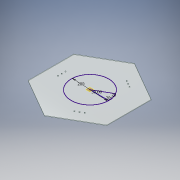
# Autodesk Inventor part: Delta_Top
Saved by Autodesk Inventor 2019 (Build 230136000, 136)
## iProperties
Created: 2019-07-06
Part Number: Delta_Top
Material: Glass
Document SubType Name: Modeling
Designer: Jorian Brusind
Density: 2.18 g/cm^3
Appearance: Clear
Author: Jorian Brusind
Autodesk Inventor part; units mm, degrees
ref_plane "YZ Plane" through (0, 0, 0) normal (1, 0, 0) x (0, 1, 0)
ref_plane "XZ Plane" through (0, 0, 0) normal (0, 1, 0) x (-1, 0, 0)
ref_plane "XY Plane" through (0, 0, 0) normal (0, 0, 1) x (1, 0, 0)
sketch "Sketch1" plane through (0, 0, 0) normal (0, 1, 0) x (-1, 0, 0)
  circle A0 centre (0, 0) radius 37.5
  line L0 (0, 0) -> (37.5, 0)
  line L1 (37.5, 0) -> (-18.75, 32.476)
  line L2 (37.5, 0) -> (102.4519, 0) construction
  line L3 (-18.75, 32.476) -> (-18.75, -32.476)
  line L4 (37.5, 0) -> (-18.75, -32.476)
  line L5 (37.5, 0) -> (37.5, 160)
  line L6 (37.5, 160) -> (37.5, 180)
  circle A1 centre (37.5, 180) radius 2.25
  circle A2 centre (37.5, 200) radius 2.25
  circle A3 centre (57.5, 180) radius 2.25
  circle A4 centre (57.5, 200) radius 2.25
  line L7 (57.5, 180) -> (67.5, 180)
  line L8 (67.5, 180) -> (67.5, 170)
  line L9 (67.5, 170) -> (7.5, 170)
  line L10 (7.5, 170) -> (7.5, 210)
  line L11 (7.5, 210) -> (67.5, 210)
  line L12 (67.5, 210) -> (67.5, 170)
  line L13 (143.4743, -91.4952) -> (178.1153, -111.4952)
  line L14 (178.1153, -111.4952) -> (148.1153, -163.4567)
  circle A5 centre (154.4551, -132.476) radius 2.25
  circle A6 centre (144.4551, -149.7965) radius 2.25
  line L15 (148.1153, -163.4567) -> (113.4743, -143.4567)
  line L16 (113.4743, -143.4567) -> (143.4743, -91.4952)
  circle A7 centre (127.1346, -139.7965) radius 2.25
  circle A8 centre (137.1346, -122.476) radius 2.25
  circle A9 centre (0, 0) radius 37.5
  line L17 (-150.9743, -78.5048) -> (-185.6153, -98.5048)
  line L18 (-185.6153, -98.5048) -> (-215.6153, -46.5433)
  circle A10 centre (-191.9551, -67.524) radius 2.25
  circle A11 centre (-201.9551, -50.2035) radius 2.25
  line L19 (-215.6153, -46.5433) -> (-180.9743, -26.5433)
  line L20 (-180.9743, -26.5433) -> (-150.9743, -78.5048)
  circle A12 centre (-184.6346, -40.2035) radius 2.25
  circle A13 centre (-174.6346, -57.524) radius 2.25
  circle A14 centre (0, 0) radius 37.5
  circle A15 centre (0, 0) radius 48
  line L21 (-215.6153, -46.5433) -> (-155.6153, -46.5433) construction
  line L22 (67.5, 210) -> (127.5, 210) construction
  line L23 (67.5, 210) -> (15, 210) construction
  line L24 (-215.6153, -46.5433) -> (-185.6153, -46.5433) construction
  line L25 (67.5, 210) -> (22.5, 210) construction
  line L26 (-215.6153, -46.5433) -> (-170.6153, -46.5433) construction
  line L27 (-215.6153, -46.5433) -> (-170.6153, -46.5433) construction
  line L28 (-18.75, -32.476) -> (-41.25, -71.4471)
  line L29 (-18.75, -32.476) -> (26.25, -32.476) construction
  line L30 (-41.25, -71.4471) -> (-84.5513, -46.4471)
  line L31 (-41.25, -71.4471) -> (2.0513, -96.4471)
  line L32 (-41.25, -71.4471) -> (8.75, -71.4471) construction
  line L33 (82.5, 0) -> (82.5, -50)
  line L34 (82.5, 0) -> (82.5, 50)
  line L35 (-41.25, 71.4471) -> (2.0513, 96.4471)
  line L36 (-41.25, 71.4471) -> (-84.5513, 46.4471)
  line L37 (-84.5513, -46.4471) -> (-84.5513, 46.4471)
  line L38 (82.5, -50) -> (2.0513, -96.4471)
  line L39 (82.5, 50) -> (2.0513, 96.4471)
  line L40 (2.0513, -240.7847) -> (-103.75, -179.7003)
  line L41 (-103.75, -179.7003) -> (-209.5513, -118.6159)
  line L42 (-209.5513, -118.6159) -> (-209.5513, 118.6159)
  line L43 (-209.5513, 118.6159) -> (-103.75, 179.7003)
  line L44 (-103.75, 179.7003) -> (2.0513, 240.7847)
  line L45 (2.0513, 240.7847) -> (207.5, 122.1688)
  line L46 (207.5, 122.1688) -> (207.5, 0)
  line L47 (207.5, 0) -> (207.5, -122.1688)
  line L48 (207.5, -122.1688) -> (2.0513, -240.7847)
  point P0 (37.5, 0)
  point P1 (-18.75, 32.476)
  point P2 (37.5, 0)
  dimension "d0" = 75
  dimension "d1" = 37.5
  dimension "d2" = 150
  dimension "d3" = 160
  dimension "d4" = 20
  dimension "d5" = 4.5
  dimension "d8" = 20
  dimension "d11" = 20
  dimension "d14" = 10
  dimension "d15" = 10
  dimension "d16" = 60
  dimension "d17" = 40
  dimension "d20" = 360
  dimension "d22" = 96
  dimension "d45" = 45
  dimension "d46" = 120
  dimension "d47" = 50
  dimension "d48" = 90
  dimension "d49" = 50
  dimension "d50" = 30
  dimension "d53" = 360
  dimension "d72" = 125
  constraints: 98 end point, 16 centre point, 14 horizontal, 6 point on circle, 5 coincident, 4 perpendicular, 4 vertical, 3 equal length, 2 parallel, 89 other
  measures "d0" diameter of A0
  measures "d1" distance of L0.start L0.end
  measures "d2" angle of L2 L1
  measures "d3" distance of L0.end L5.end
  measures "d4" distance of L5.end L6.end
  measures "d5" diameter of A1
  measures "d8" distance of A1.centre A2.centre
  measures "d11" distance of A1.centre L7.start
  measures "d14" distance of L7.start L7.end
  measures "d15" distance of L7.end L8.end
  measures "d16" distance of L10.end L11.end
  measures "d17" distance of L9.end L10.end
  measures "d22" diameter of A15
  measures "d45" distance of L28.start L28.end
  measures "d46" angle of L28 L29
  measures "d47" distance of L28.end L30.end
  measures "d48" angle of L28 L30
  measures "d49" distance of L28.end L31.end
  measures "d50" angle of L31 L32
  measures "d72" distance between parallel lines of L38 L48
ref_plane "Work Plane2" through (0, 3, 0) normal (0, 1, 0) x (1, 0, 0)
ref_plane "Work Plane1" through (0, 3, 0) normal (0, 1, 0) x (1, 0, 0)
extrude "Extrusion8" add sketch "Sketch1" along normal blind 3 contours L1 A0 | L5 A15 L28 A0 | L4 L3 L1 | A0 L4 | A0 L28 A15 L5 | L3 A0 | A15 L28 L30 L37 L36 L35 L39 L5 | L5 L39 L34 L33 L38 L31 L28 A15 | A1 | A2 | A3 | A4 | L12 L45 L46 L47 L48 L14 L13 L16 L15 L40 L41 L42 L18 L17 L20 L19 L43 L44 L11 L10 L9 L8 | L8 L9 L10 L11 L45 L12 | L48 L15 L16 L13 L14 | L19 L20 L17 L18 L42 | A5 | A6 | A7 | A8 | A10 | A11 | A12 | A13
sketch "Sketch4" plane through (0, 3, 0) normal (0, 1, 0) x (1, 0, 0)
  line L0 (0, 0) -> (-150, 0)
  circle A0 centre (0, 0) radius 2.5
  line L1 (-150, 0) -> (-150, -19.995)
  circle A1 centre (-150, -19.995) radius 2.5
  line L2 (-150, 0) -> (-150, 19.995)
  circle A2 centre (-150, 19.995) radius 2.5
  circle A3 centre (-150, 0) radius 2.5
  dimension "d79" = 150
  dimension "d80" = 5
  dimension "d81" = 19.995
  dimension "d82" = 5
  dimension "d83" = 19.995
  dimension "d84" = 5
  dimension "d90" = 5
  constraints: 6 end point, 4 centre point, 4 coincident, 2 vertical, 1 horizontal
  measures "d79" distance of L0.start L0.end
  measures "d80" diameter of A0
  measures "d81" distance of L0.end L1.end
  measures "d82" diameter of A1
  measures "d83" distance of L0.end L2.end
  measures "d84" diameter of A2
  measures "d90" diameter of A3
extrude "Extrusion10" cut sketch "Sketch4" against normal blind 3
pattern_circular "Circular Pattern2" count 3 over 360 about axis through (0, 3, 0) along (0, -1, 0) of "Extrusion10"
sketch "Sketch5" plane through (0, 3, 0) normal (0, 1, 0) x (1, 0, 0)
  circle A0 centre (0, 0) radius 100
  circle A1 centre (0, 0) radius 2.5 projected
  line L0 (0, 0) -> (100, 0)
  line L1 (100, 0) -> (100, 20)
  line L2 (0, 0) -> (86.6025, 50)
  line L3 (0, 0) -> (100, 0) construction
  line L4 (86.6025, 50) -> (96.6025, 32.6795)
  dimension "d96" = 200
  dimension "d97" = 20
  dimension "d98" = 30
  dimension "d99" = 20
  constraints: 10 end point, 2 horizontal, 2 point on circle, 2 tangent, 1 centre point, 1 coincident, 1 equal length, 1 perpendicular
  measures "d96" diameter of A0
  measures "d97" distance of L0.end L1.end
  measures "d98" angle of L3 L2
  measures "d99" distance of L2.end L4.end
body "Solid5"
